Multimeter Case (Autodesk Fusion 360 design; units mm, degrees)
Autodesk Fusion 360 part; units mm, degrees
sketch "Body" plane through (0, 0, 0) normal (0, 1, 0) x (1, 0, 0)
  line L0 (0, 0) -> (59.4, 0)
  line L1 (59.4, 0) -> (59.4, 41.2)
  line L2 (59.4, 41.2) -> (0, 41.2)
  line L3 (0, 41.2) -> (0, 0)
  line L4 (2, 39.2) -> (57.4, 39.2)
  line L5 (57.4, 39.2) -> (57.4, 2)
  line L6 (57.4, 2) -> (2, 2)
  line L7 (2, 2) -> (2, 39.2)
  dimension "d1" = 59.4
  dimension "d2" = 41.2
  dimension "d3" = 2
  dimension "d4" = 2
  dimension "d5" = 2
  dimension "d6" = 2
  constraint horizontal L0
  constraint vertical L1
  constraint horizontal L2
  constraint vertical L3
  constraint coincident L0.start L3.end
  constraint horizontal L4
  constraint vertical L5
  constraint horizontal L6
  constraint vertical L7
  measures "d1" horizontal distance of L1.end L2.end
  measures "d2" vertical distance of L0.end L1.end
  measures "d3" distance of L2 L4
  measures "d4" distance of L0 L6
  measures "d5" distance of L3 L7
  measures "d6" distance of L1 L5
extrude "Extrude1" add sketch "Body" along normal blind 2 contours L0 L1 L2 L3 | L4 L5 L6 L7 makes body 1
extrude "Extrude2" add sketch "Body" along normal blind 32 bodies 1
sketch "Back Holes" plane through (0, 0, 0) normal (0, 0, 1) x (1, 0, 0)
  line L0 (13.5, 20.5) -> (26.5, 20.5)
  line L1 (26.5, 20.5) -> (26.5, 13)
  line L2 (26.5, 13) -> (13.5, 13)
  line L3 (13.5, 13) -> (13.5, 20.5)
  line L4 (0, 0) -> (59.4, 0)
  line L5 (0, 0) -> (0, 32)
  line L6 (31.4, 27) -> (44.4, 27)
  line L7 (44.4, 27) -> (44.4, 24)
  line L8 (44.4, 24) -> (31.4, 24)
  line L9 (31.4, 24) -> (31.4, 27)
  line L10 (59.4, 0) -> (59.4, 32)
  line L11 (0, 32) -> (59.4, 32)
  dimension "d11" = 13
  dimension "d13" = 13
  dimension "d14" = 13.5
  dimension "d15" = 13
  dimension "d16" = 3
  dimension "d36" = 15
  dimension "d37" = 5
  constraint horizontal L0
  constraint vertical L1
  constraint horizontal L2
  constraint vertical L3
  constraint horizontal L6
  constraint vertical L7
  constraint horizontal L8
  constraint vertical L9
  measures "d11" horizontal distance of L0.start L0.end
  measures "d13" distance of L2 L4
  measures "d14" distance of L3 L5
  measures "d15" distance of L6.start L6.end
  measures "d16" distance of L6.start L8.end
  measures "d36" distance of L7 L10
  measures "d37" distance of L6 L11
extrude "Extrude3" cut sketch "Back Holes" against normal blind 5 contours L0 L1 L2 L3 | L6 L7 L8 L9 bodies 1
sketch "Front Holes" plane through (0, 0, 0) normal (0, 0, 1) x (1, 0, 0)
  circle A0 centre (49.4, 22) radius 5.5
  line L0 (0, 0) -> (59.4, 0)
  line L1 (0, 0) -> (0, 32)
  line L2 (59.4, 0) -> (59.4, 32)
  line L3 (0, 32) -> (59.4, 32)
  dimension "d22" = 11
  dimension "d38" = 10
  dimension "d39" = 10
  measures "d22" diameter of A0
  measures "d38" distance of A0.centre L2
  measures "d39" distance of A0.centre L3
extrude "Extrude4" cut sketch "Front Holes" against normal blind 10 from surface at -35 contours A0 bodies 1
sketch "Sketch4" plane through (0, 0, 0) normal (0, 1, 0) x (1, 0, 0)
  line L0 (3.5, 37.7) -> (55.9, 37.7)
  line L1 (55.9, 37.7) -> (55.9, 3.5)
  line L2 (55.9, 3.5) -> (3.5, 3.5)
  line L3 (3.5, 3.5) -> (3.5, 37.7)
  line L4 (2, 39.2) -> (57.4, 39.2)
  line L5 (57.4, 39.2) -> (57.4, 2)
  line L6 (57.4, 2) -> (2, 2)
  line L7 (2, 2) -> (2, 39.2)
  dimension "d28" = 1.5
  dimension "d29" = 1.5
  dimension "d30" = 1.5
  dimension "d31" = 1.5
  constraint horizontal L0
  constraint vertical L1
  constraint horizontal L2
  constraint vertical L3
  measures "d28" distance of L0 L4
  measures "d29" distance of L1 L5
  measures "d30" distance of L2 L6
  measures "d31" distance of L3 L7
extrude "Extrude5" add sketch "Body" along normal blind 2 separate body contours L0 L1 L2 L3 | L4 L5 L6 L7 makes body 2
extrude "Extrude6" add sketch "Sketch4" against normal blind 1.5 bodies 2
copy_body "Body->Comp1" bodies 1 removing the originals makes body 3 in component "Case"
copy_body "Body->Comp2" bodies 2 removing the originals makes body 4 in component "Lid"
sketch "Sketch5" plane through (0, 0, 0) normal (0, 1, 0) x (1, 0, 0)
  line L0 (57.4, 39.2) -> (54.4, 39.2)
  line L1 (54.4, 39.2) -> (54.4, 34.2)
  line L2 (54.4, 34.2) -> (57.4, 34.2)
  line L3 (57.4, 34.2) -> (57.4, 39.2)
  line L4 (57.4, 2) -> (54.4, 2)
  line L5 (54.4, 2) -> (54.4, 7)
  line L6 (54.4, 7) -> (57.4, 7)
  line L7 (57.4, 7) -> (57.4, 2)
  line L8 (2, 2) -> (5, 2)
  line L9 (5, 2) -> (5, 7)
  line L10 (5, 7) -> (2, 7)
  line L11 (2, 7) -> (2, 2)
  line L12 (2, 39.2) -> (7, 39.2)
  line L13 (7, 39.2) -> (7, 36.2)
  line L14 (7, 36.2) -> (2, 36.2)
  line L15 (2, 36.2) -> (2, 39.2)
  point P0 (57.4, 39.2)
  point P1 (57.4, 2)
  point P2 (2, 2)
  point P3 (2, 39.2)
  dimension "d40" = 3
  dimension "d41" = 5
  dimension "d42" = 3
  dimension "d43" = 5
  dimension "d44" = 5
  dimension "d45" = 3
  dimension "d46" = 5
  dimension "d47" = 3
  constraint horizontal L0
  constraint vertical L1
  constraint horizontal L2
  constraint vertical L3
  constraint coincident P0 L0.start
  constraint horizontal L4
  constraint vertical L5
  constraint horizontal L6
  constraint vertical L7
  constraint coincident P1 L4.start
  constraint horizontal L8
  constraint vertical L9
  constraint horizontal L10
  constraint vertical L11
  constraint coincident P2 L8.start
  constraint horizontal L12
  constraint vertical L13
  constraint horizontal L14
  constraint vertical L15
  constraint coincident P3 L12.start
  measures "d40" distance of P0 L0.end
  measures "d41" distance of P0 L2.end
  measures "d42" distance of P1 L4.end
  measures "d43" distance of P1 L6.end
  measures "d44" distance of P2 L10.end
  measures "d45" distance of P2 L8.end
  measures "d46" distance of P3 L12.end
  measures "d47" distance of P3 L14.end
extrude "Extrude1'" add sketch "Sketch5" along normal blind 4 bodies 3 in component "Case"
extrude "Extrude1''" add 1 faces at (20.9667, -1.5, -38.7) along direction (0, -1, 0) blind 1.5 on bodies 4 bodies 4 in component "Lid"
component "NodeMCU v1" placed x (1, 0, 0) y (0, 1, 0) z (0, 0, 1) at (0, 0, 0)
component "Case" placed x (1, 0, 0) y (0, 1, 0) z (0, 0, 1) at (0, 0, 0)
component "Lid" placed x (1, 0, 0) y (0, 1, 0) z (0, 0, 1) at (0, 0, 0)
named bodies: "Case", "Lid"
